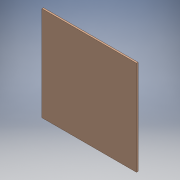
# Autodesk Inventor part: base_plank
Saved by Autodesk Inventor 2018 (Build 220112000, 112)
## iProperties
Created: 2018-09-09
Part Number: base_plank
Material: Generic
Document SubType Name: Modeling
Designer: Fredy Espana C
Density: 1 g/cm^3
Appearance: Default
Author: Fredy Espana C
Autodesk Inventor part; units mm, degrees
ref_plane "YZ Plane" through (0, 0, 0) normal (1, 0, 0) x (0, 1, 0)
ref_plane "XZ Plane" through (0, 0, 0) normal (0, 1, 0) x (-1, 0, 0)
ref_plane "XY Plane" through (0, 0, 0) normal (0, 0, 1) x (1, 0, 0)
sketch "Sketch1" plane through (0, 0, 0) normal (0, 1, 0) x (-1, 0, 0)
  line L0 (0, 0) -> (360, 0)
  line L1 (360, 0) -> (360, -360)
  line L2 (360, -360) -> (0, -360)
  line L3 (0, -360) -> (0, 0)
  dimension "d0" = 360
  dimension "d1" = 360
  constraints: 8 end point, 2 parallel, 1 horizontal, 1 perpendicular
  measures "d0" distance of L2.end L0.start
  measures "d1" distance of L0.start L0.end
extrude "Extrusion1" add sketch "Sketch1" along normal blind 6
body "Solid1"
